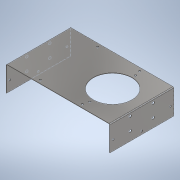
# Autodesk Inventor part: tapa_v7
Saved by Autodesk Inventor 2020.3 (Build 243373000, 373)
## iProperties
Created: 2020-06-30
Part Number: tapa_v7
Material: Steel, Carbon
Document SubType Name: Sheet Metal
Designer: Bruno
Density: 7.85 g/cm^3
Sheet Metal Rule: Default_mm
Appearance: Semi-Polished
Author: Bruno
Autodesk Inventor part; units mm, degrees
ref_plane "YZ Plane" through (0, 0, 0) normal (1, 0, 0) x (0, 1, 0)
ref_plane "XZ Plane" through (0, 0, 0) normal (0, 1, 0) x (-1, 0, 0)
ref_plane "XY Plane" through (0, 0, 0) normal (0, 0, 1) x (1, 0, 0)
sketch "Sketch1" plane through (0, 0, 0) normal (0, 1, 0) x (-1, 0, 0)
  line L0 (0, 0) -> (252, 0)
  line L1 (252, 0) -> (252, -155)
  line L2 (252, -155) -> (0, -155)
  line L3 (0, -155) -> (0, 0)
  dimension "d0" = 252
  dimension "d1" = 155
  measures "d0" distance of L1.end L2.end
  measures "d1" distance of L0.end L1.end
extrude "Plate1" add sketch "Sketch1" along normal blind 1
sketch "Sketch2" plane through (-1, 1, 0) normal (1, 0, 0) x (0, 1, 0)
  line L0 (0, -155) -> (0, 0)
  line L1 (0, 0) -> (-61, 0)
  line L2 (-61, 0) -> (-61, -155)
  line L3 (-61, -155) -> (0, -155)
  constraints: 6 end point, 1 horizontal, 1 perpendicular, 1 vertical
edge flange "Flange1" height 61 angle 90 thickness 1 bend radius 1 thickness toward (1, 0, 0) relief straight relief width 1 relief depth 0.5 edges at (0, 0, -77.5) wall of the first edge with corners at (-1, 1, -155) (-1, 1, 0) (-1, -60, 0) (-1, -60, -155)
bend "Bend1"
corner "Corner1"
sketch "Sketch3" plane through (-251, 1, -155) normal (-1, 0, 0) x (0, -1, 0)
  line L0 (0, 155) -> (0, 0)
  line L1 (0, 0) -> (61, 0)
  line L2 (61, 0) -> (61, 155)
  line L3 (61, 155) -> (0, 155)
  constraints: 6 end point, 1 horizontal, 1 perpendicular, 1 vertical
edge flange "Flange2" height 61 angle 90 thickness 1 bend radius 1 thickness toward (-1, 0, 0) relief straight relief width 1 relief depth 0.5 edges at (-252, 0, -77.5) wall of the first edge with corners at (-251, 1, 0) (-251, 1, -155) (-251, -60, -155) (-251, -60, 0)
bend "Bend2"
corner "Corner2"
sketch "Sketch4" plane through (0, 1, 0) normal (0, 1, 0) x (1, 0, 0)
  line L0 (0, 155) -> (0, 0) projected
  line L1 (0, 0) -> (0, 77.5)
  line L2 (0, 77.5) -> (-71, 77.5)
  circle A0 centre (-71, 77.5) radius 47
  line L3 (-71, 77.5) -> (-71, 133) construction
  line L4 (-71, 77.5) -> (-71, 22) construction
  circle A1 centre (-71, 133) radius 2.25
  circle A2 centre (-71, 22) radius 2.25
  dimension "d23" = 77.5
  dimension "d24" = 71
  dimension "d25" = 94
  dimension "d26" = 55.5
  dimension "d27" = 55.5
  dimension "d28" = 4.5
  dimension "d29" = 4.5
  constraints: 8 end point, 3 centre point, 3 coincident, 2 vertical, 1 midpoint, 1 perpendicular
  measures "d23" distance of L0.end L1.end
  measures "d24" distance of L1.end L2.end
  measures "d25" diameter of A0
  measures "d26" distance of L3.start L3.end
  measures "d27" distance of L3.start L4.end
  measures "d28" diameter of A1
  measures "d29" diameter of A2
extrude "Extrusion1" cut sketch "Sketch4" against normal through all
sketch "Sketch5" plane through (0, 1, 0) normal (0, 1, 0) x (1, 0, 0)
  line L0 (-252, 0) -> (-252, 155) projected
  line L1 (0, 155) -> (0, 0) projected
  line L2 (-250, 155) -> (-2, 155) projected
  line L3 (-2, 0) -> (-250, 0) projected
  point P0 (-177, 147)
  point P1 (-75, 147)
  point P2 (-177, 8)
  point P3 (-75, 8)
  dimension "d32" = 75
  dimension "d33" = 75
  dimension "d34" = 8
  dimension "d35" = 8
  constraints: 2 horizontal alignment, 2 vertical alignment
  measures "d32" distance from line of L0 point (-177, 147)
  measures "d33" distance from line of point (-75, 147) L1
  measures "d34" distance from line of L2 point (-177, 147)
  measures "d35" distance from line of L3 point (-177, 8)
hole "Hole1" at (-177, 1, -147) at (-75, 1, -147) at (-177, 1, -8) at (-75, 1, -8) direction (0, -1, 0) diameter 4.5 end through all
sketch "Sketch6" plane through (0, -60, 0) normal (1, 0, 0) x (0, 0, -1)
  line L0 (0, 0) -> (0, 59) projected
  line L1 (155, 0) -> (0, 0) projected
  line L2 (155, 59) -> (155, 0) projected
  point P0 (0, 60)
  point P1 (8, 24)
  point P2 (77.5, 7)
  point P3 (147, 24)
  dimension "d43" = 77.5
  dimension "d44" = 7
  dimension "d45" = 8
  dimension "d46" = 8
  dimension "d47" = 24
  dimension "d48" = 24
  measures "d43" distance from line of L0 point (77.5, 7)
  measures "d44" distance from line of point (77.5, 7) L1
  measures "d45" distance from line of point (8, 24) L0
  measures "d46" distance from line of point (147, 24) L2
  measures "d47" distance from line of L1 point (8, 24)
  measures "d48" distance from line of L1 point (147, 24)
hole "Hole2" at (0, -36, -8) at (0, -53, -77.5) at (0, -36, -147) direction (-1, 0, 0) diameter 4.5 end through all
sketch "Sketch7" plane through (0, -60, 0) normal (1, 0, 0) x (0, 0, -1)
  line L0 (155, 60) -> (0, 60) projected
  line L1 (0, 59) -> (155, 59) projected
  line L2 (77.5, 59) -> (42.5, 59)
  line L3 (42.5, 59) -> (42.5, 14)
  line L4 (42.5, 14) -> (112.5, 14)
  line L5 (112.5, 14) -> (112.5, 59)
  point P0 (49.5, 52)
  point P1 (49.5, 21)
  point P2 (105.5, 21)
  point P3 (105.5, 52)
  dimension "d57" = 35
  dimension "d58" = 45
  dimension "d59" = 70
  dimension "d60" = 7
  dimension "d61" = 7
  dimension "d62" = 7
  dimension "d63" = 7
  constraints: 8 end point, 3 perpendicular, 2 horizontal alignment, 2 point on line, 2 vertical alignment, 1 midpoint
  measures "d57" distance of L2.start L2.end
  measures "d58" distance of L2.end L3.end
  measures "d59" distance of L3.end L4.end
  measures "d60" distance from line of L3 point (49.5, 52)
  measures "d61" distance from line of L5 point (105.5, 52)
  measures "d62" distance from line of L1 point (49.5, 52)
  measures "d63" distance from line of L4 point (49.5, 21)
hole "Hole3" at (0, -8, -49.5) at (0, -39, -49.5) at (0, -39, -105.5) at (0, -8, -105.5) direction (-1, 0, 0) diameter 6 depth 1 tip angle 118
equation "\"d33\" = d32"
equation "\"d34\" = d35"
equation "\"d41\" = Thickness"
equation "\"d46\" = d45"
equation "\"d48\" = d47"
equation "\"d54\" = Thickness"
equation "\"d61\" = d60"
equation "\"d63\" = d62"
equation "\"d69\" = Thickness"
equation "\"d2\" = Thickness"
equation "\"d3\" = BendReliefWidth"
equation "\"d4\" = BendReliefDepth"
equation "\"d5\" = MinimumRemnant"
equation "\"d6\" = TransitionRadius"
equation "\"d9\" = BendRadius"
equation "\"d10\" = CornerReliefSize"
equation "\"d11\" = GapSize"
equation "\"d12\" = JacobiRadiusSize"
equation "\"d13\" = BendReliefWidth"
equation "\"d14\" = BendReliefDepth"
equation "\"d15\" = MinimumRemnant"
equation "\"d16\" = TransitionRadius"
equation "\"d19\" = BendRadius"
equation "\"d20\" = CornerReliefSize"
equation "\"d21\" = GapSize"
equation "\"d22\" = JacobiRadiusSize"
equation "\"BendRadius\" = Thickness"
equation "\"BendReliefWidth\" = Thickness"
equation "\"BendReliefDepth\" = 0.5 * Thickness"
equation "\"CornerReliefSize\" = 4 * Thickness"
equation "\"MinimumRemnant\" = 2 * Thickness"
equation "\"TransitionRadius\" = BendRadius"
equation "\"JacobiRadiusSize\" = BendRadius"
equation "\"GapSize\" = Thickness"
equation "\"Thickness\" = 1"
body "Solid1"
